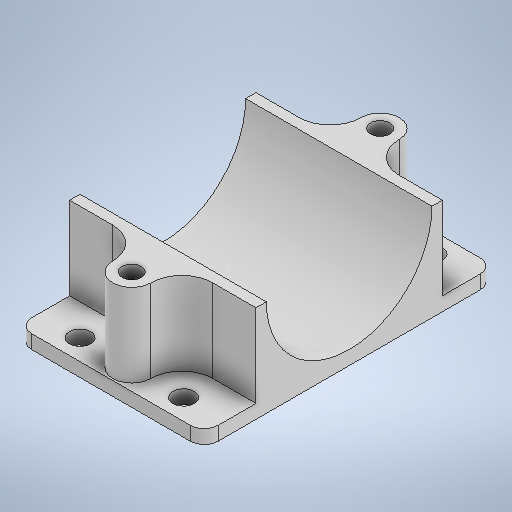
# Autodesk Inventor part: daisen_moto_parts1
Saved by Autodesk Inventor 2025.2 (Build 292293000, 293)
## iProperties
Created: 2025-01-13
Part Number: daisen_moto_parts1
Material: 一般
Document SubType Name: Modeling
Designer: mahhy
Density: 1 g/cm^3
Appearance: 既定
Author: mahhy
Autodesk Inventor part; units mm, degrees
ref_plane "YZ Plane" through (0, 0, 0) normal (1, 0, 0) x (0, 1, 0)
ref_plane "XZ Plane" through (0, 0, 0) normal (0, 1, 0) x (-1, 0, 0)
ref_plane "XY Plane" through (0, 0, 0) normal (0, 0, 1) x (1, 0, 0)
sketch "スケッチ1" plane through (0, 0, 0) normal (0, 1, 0) x (-1, 0, 0)
  line L0 (2, 0) -> (25, 0)
  line L1 (27, -2) -> (27, -40)
  line L2 (25, -42) -> (2, -42)
  line L3 (0, -40) -> (0, -2)
  arc A0 (27, -2) -> (25, 0) centre (25, -2) ccw
  arc A1 (25, -42) -> (27, -40) centre (25, -40) ccw
  arc A2 (2, 0) -> (0, -2) centre (2, -2) ccw
  arc A3 (0, -40) -> (2, -42) centre (2, -40) ccw
  point P0 (0, 0)
  point P1 (27, -42)
  point P2 (27, 0)
  point P3 (0, -42)
  dimension "d0" = 27
  dimension "d1" = 42
  dimension "d2" = 2
  constraints: 8 end point, 8 point on circle, 8 point on line, 8 tangent, 4 centre point, 3 equal radius, 2 parallel, 1 horizontal, 1 perpendicular
  measures "d0" distance of point (27, -42) point (0, -42)
  measures "d1" distance of point (27, 0) point (27, -42)
  measures "d2" radius of A0
extrude "押し出し1" add sketch "スケッチ1" along normal blind 2
sketch "スケッチ2" plane through (0, 2, 0) normal (0, 1, 0) x (1, 0, 0)
  line L0 (-27, 40) -> (-27, 2) projected
  line L1 (0, 2) -> (0, 40) projected
  line L2 (-2, 42) -> (-25, 42) projected
  line L3 (-25, 0) -> (-2, 0) projected
  point P0 (0, 0)
  point P1 (-21, 39)
  point P2 (-6, 39)
  point P3 (-21, 3)
  point P4 (-6, 3)
  dimension "d5" = 6
  dimension "d6" = 6
  dimension "d7" = 6
  dimension "d8" = 6
  dimension "d9" = 3
  dimension "d10" = 3
  dimension "d11" = 3
  dimension "d12" = 3
  measures "d5" distance from line of L0 point (-21, 39)
  measures "d6" distance from line of L1 point (-6, 39)
  measures "d7" distance from line of L1 point (-6, 3)
  measures "d8" distance from line of L0 point (-21, 3)
  measures "d9" distance from line of L2 point (-6, 39)
  measures "d10" distance from line of L2 point (-21, 39)
  measures "d11" distance from line of L3 point (-21, 3)
  measures "d12" distance from line of point (-6, 3) L3
hole "穴1" at (-21, 2, -39) at (-6, 2, -39) at (-21, 2, -3) at (-6, 2, -3) direction (0, -1, 0) diameter 3.1 end through all
sketch "スケッチ3" plane through (0, 2, 0) normal (0, 1, 0) x (1, 0, 0)
  line L0 (-27, 40) -> (-27, 2) projected
  line L1 (-27, 34.5) -> (0, 34.5)
  line L2 (0, 34.5) -> (0, 7.5)
  line L3 (0, 7.5) -> (-27, 7.5)
  line L4 (-27, 7.5) -> (-27, 34.5)
  line L5 (0, 2) -> (0, 40) projected
  circle A0 centre (-13.5, 3) radius 2.75
  circle A1 centre (-13.5, 39) radius 2.75
  arc A2 (-20.75, 34.5) -> (-16.25, 39) centre (-20.75, 39) ccw
  arc A3 (-10.75, 39) -> (-6.25, 34.5) centre (-6.25, 39) ccw
  line L6 (-16.25, 3) -> (-20.75, 3)
  line L7 (-10.75, 3) -> (-6.25, 3)
  arc A4 (-16.25, 3) -> (-20.75, 7.5) centre (-20.75, 3) ccw
  arc A5 (-6.25, 7.5) -> (-10.75, 3) centre (-6.25, 3) ccw
  point P0 (0, 0)
  point P1 (0, 21)
  point P2 (0, 21)
  dimension "d20" = 27
  dimension "d21" = 27
  dimension "d22" = 0
  dimension "d23" = 5.5
  dimension "d24" = 5.5
  dimension "d25" = 4.5
  dimension "d27" = 4.5
  dimension "d29" = 4.5
  dimension "d30" = 4.5
  constraints: 13 point on circle, 12 end point, 6 centre point, 4 point on line, 3 horizontal, 2 coincident, 2 midpoint, 2 parallel, 1 perpendicular
  measures "d20" distance of L2.end L3.end
  measures "d21" distance of L1.end L2.end
  measures "d22" distance of point (0, 21) point (0, 21)
  measures "d23" diameter of A0
  measures "d24" diameter of A1
  measures "d25" distance from line of L1 A1.centre
  measures "d27" radius of A2
  measures "d29" distance of L6.start L6.end
  measures "d30" distance of L7.start L7.end
extrude "押し出し2" add sketch "スケッチ3" along normal blind 12
sketch "スケッチ4" plane through (0, 0, -2) normal (1, 0, 0) x (0, 0, -1)
  line L0 (32.5, 14) -> (5.5, 14) projected
  circle A0 centre (19, 14) radius 12
  point P0 (-2, 0)
  point P1 (7, 14)
  point P2 (31, 14)
  dimension "d33" = 24
  constraints: 1 centre point, 1 midpoint
  measures "d33" diameter of A0
extrude "押し出し3" cut sketch "スケッチ4" against normal through all contours A0 L0 picked at (15.4582, 12.1411)
sketch "スケッチ5" plane through (0, 14, 0) normal (0, 1, 0) x (1, 0, 0)
  arc A0 (-10.75, 39) -> (-16.25, 39) centre (-13.5, 39) ccw projected
  arc A1 (-16.25, 3) -> (-10.75, 3) centre (-13.5, 3) ccw projected
  point P0 (0, 0)
  constraints: 2 coincident
hole "穴2" at (-13.5, 14, -39) at (-13.5, 14, -3) direction (0, -1, 0) diameter 2.8 end through all
